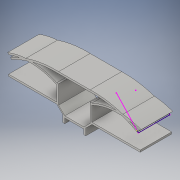
# Autodesk Inventor part: Test
Saved by Autodesk Inventor 2016 (Build 200138000, 138)
## iProperties
Created: 2015-09-24
Part Number: Test
Material: Generic
Document SubType Name: Modeling
Designer: fei
Density: 1 g/cm^3
Appearance: Default
Author: fei
Autodesk Inventor part; units mm, degrees
ref_plane "YZ Plane" through (0, 0, 0) normal (1, 0, 0) x (0, 1, 0)
ref_plane "XZ Plane" through (0, 0, 0) normal (0, 1, 0) x (-1, 0, 0)
ref_plane "XY Plane" through (0, 0, 0) normal (0, 0, 1) x (1, 0, 0)
sketch "Sketch1" plane through (0, 0, 0) normal (1, 0, 0) x (0, 1, 0)
  line L0 (38.1, 647.7) -> (-38.1, 647.7)
  line L1 (-38.1, 647.7) -> (-38.1, -647.7)
  line L2 (-38.1, -647.7) -> (38.1, -647.7)
  line L3 (38.1, -647.7) -> (38.1, 647.7)
  line L4 (0, 0) -> (420.0175, 0) construction
  point P0 (0, 647.7)
  dimension "d0" = 76.2
  dimension "d1" = 1295.4
  dimension "d2" = 647.7
  constraints: 10 end point, 2 horizontal, 2 parallel, 1 midpoint, 1 perpendicular, 1 vertical alignment
  measures "d0" distance of L1.end L2.end
  measures "d1" distance of L2.end L0.start
  measures "d2" distance between parallel lines of L0 L4
extrude "Extrusion1" add sketch "Sketch1" along normal blind 469.9
sketch "Sketch2" plane through (0, -38.1, -647.7) normal (0, -1, 0) x (1, 0, 0)
  line L0 (0, 0) -> (469.9, 0) projected
  line L1 (469.9, 1295.4) -> (393.7, 1295.4)
  line L2 (393.7, 1295.4) -> (393.7, 0)
  line L3 (393.7, 0) -> (469.9, 0)
  line L4 (469.9, 0) -> (469.9, 1295.4)
  point P0 (0, 647.7)
  dimension "d5" = 76.2
  constraints: 8 end point, 2 parallel, 1 horizontal, 1 perpendicular, 1 point on line
  measures "d5" distance of L2.end L0.end
extrude "Extrusion2" add sketch "Sketch2" along normal blind 203.2
sketch "Sketch3" plane through (0, 38.1, 647.7) normal (0, 1, 0) x (1, 0, 0)
  line L0 (469.9, 1295.4) -> (469.9, 0) projected
  line L1 (393.7, 0) -> (393.7, 1295.4) projected
  line L2 (469.9, 1295.4) -> (393.7, 1295.4)
  line L3 (393.7, 1295.4) -> (393.7, 0)
  line L4 (393.7, 0) -> (469.9, 0)
  line L5 (469.9, 0) -> (469.9, 1295.4)
  point P0 (0, 647.7)
  constraints: 8 end point, 2 parallel, 1 horizontal, 1 perpendicular
sketch "Sketch4" plane through (0, 0, 0) normal (0, 0, 1) x (1, 0, 0)
  line L0 (0, 38.1) -> (469.9, 38.1) projected
  line L1 (431.8, 38.1) -> (685.8, 292.1)
  point P0 (0, 0)
  dimension "d10" = 135
  dimension "d11" = 38.1
  dimension "d12" = 254
  constraints: 2 end point, 1 point on line
  measures "d10" angle of L0 L1
  measures "d11" distance of L0.end L1.start
  measures "d12" horizontal distance of L1.start L1.end
sweep "Sweep1" add profiles "Sketch3" path "Sketch4" path curves L1
sketch "Sketch5" plane through (647.7, 292.1, -647.7) normal (0, 1, 0) x (1, 0, 0)
  line L0 (76.2, -1295.4) -> (76.2, 0) projected
  line L1 (-254, -1295.4) -> (0, -1295.4) projected
  line L2 (76.2, 0) -> (0, 0)
  line L3 (0, 0) -> (0, -1295.4)
  line L4 (0, -1295.4) -> (76.2, -1295.4)
  line L5 (76.2, -1295.4) -> (76.2, 0)
  point P0 (-647.7, -647.7)
  constraints: 8 end point, 2 parallel, 1 horizontal, 1 perpendicular
extrude "Extrusion3" add sketch "Sketch5" along normal blind 76.2
sketch "Sketch6" plane through (723.9, 292.1, -647.7) normal (1, 0, 0) x (0, 0, -1)
  line L0 (-1295.4, 0) -> (-1295.4, 76.2) projected
  line L1 (0, -254) -> (0, 0) projected
  line L2 (-1295.4, 76.2) -> (0, 76.2)
  line L3 (0, 76.2) -> (0, 0)
  line L4 (0, 0) -> (-1295.4, 0)
  line L5 (-1295.4, 0) -> (-1295.4, 76.2)
  point P0 (-647.7, -292.1)
  constraints: 8 end point, 2 parallel, 1 horizontal, 1 perpendicular
extrude "Extrusion4" add sketch "Sketch6" along normal blind 1981.2
sketch "Sketch7" plane through (647.7, 368.3, -647.7) normal (0, 1, 0) x (1, 0, 0)
  line L0 (0, 0) -> (0, -1295.4) projected
  line L1 (0, 0) -> (76.2, 0)
  line L2 (76.2, 0) -> (76.2, -1295.4)
  line L3 (76.2, -1295.4) -> (0, -1295.4)
  line L4 (0, -1295.4) -> (0, 0)
  point P0 (-647.7, -647.7)
  dimension "d19" = 76.2
  constraints: 8 end point, 2 parallel, 1 horizontal, 1 perpendicular
  measures "d19" distance of L0.start L1.end
extrude "Extrusion5" add sketch "Sketch7" along normal blind 609.6
sketch "Sketch8" plane through (0, 0, 0) normal (0, 0, 1) x (1, 0, 0)
  line L0 (647.7, 977.9) -> (723.9, 977.9) projected
  arc A0 (2705.1, 1079.5) -> (685.8, 977.9) centre (1812.5424, -1298.512) ccw
  line L1 (723.9, 977.9) -> (2746.3916, 977.9) construction
  line L2 (723.9, 368.3) -> (2705.1, 368.3) construction
  line L3 (2705.1, 368.3) -> (2705.1, 1575.1367) construction
  point P0 (0, 0)
  dimension "d22" = 2540
  dimension "d23" = 101.6
  constraints: 4 end point, 2 point on circle, 1 centre point, 1 horizontal, 1 midpoint, 1 point on line, 1 vertical
  measures "d22" radius of A0
  measures "d23" distance from line of L1 A0.start
sketch "Sketch9" plane through (647.7, 977.9, -647.7) normal (0, 1, 0) x (1, 0, 0)
  line L0 (0, 0) -> (0, -1295.4) projected
  line L1 (-177.8, -1295.4) -> (76.2, -1295.4) projected
  line L2 (0, 0) -> (76.2, 0)
  line L3 (76.2, 0) -> (76.2, -1295.4)
  line L4 (76.2, -1295.4) -> (0, -1295.4)
  line L5 (0, -1295.4) -> (0, 0)
  point P0 (-647.7, -647.7)
  constraints: 8 end point, 2 parallel, 1 horizontal, 1 perpendicular
sketch "Sketch12" plane through (0, 0, 0) normal (1, 0, 0) x (0, 1, 0)
  line L0 (1487.2171, -647.7) -> (1411.0171, -647.7)
  line L1 (1411.0171, -647.7) -> (1411.0171, 647.7)
  line L2 (1411.0171, 647.7) -> (1487.2171, 647.7)
  line L3 (1487.2171, 647.7) -> (1487.2171, -647.7)
  line L4 (876.3, -647.7) -> (1157.0171, -647.7) construction
  line L5 (876.3, 647.7) -> (1157.0171, 647.7) construction
  line L6 (1157.0171, -647.7) -> (1157.0171, 647.7) construction
  point P0 (0, 0)
  point P1 (1005.7223, -647.7)
  point P2 (1005.7223, 647.7)
  dimension "d26" = 1295.4
  dimension "d27" = 76.2
  dimension "d28" = 254
  dimension "d29" = 647.7
  constraints: 10 end point, 2 parallel, 1 horizontal, 1 perpendicular, 1 vertical
  measures "d26" distance of L2.end L0.start
  measures "d27" distance of L0.start L0.end
  measures "d28" distance between parallel lines of L6 L1
  measures "d29" distance from line of point (0, 0) L0
extrude "Extrusion6" add sketch "Sketch12" along normal blind 647.7
sketch "Sketch13" plane through (0, 0, 0) normal (0, 0, 1) x (1, 0, 0)
  line L0 (2577.4706, 1005.7223) -> (2629.5294, 950.0777) projected
  line L1 (647.7, 1411.0171) -> (647.7, 1487.2171) projected
  arc A0 (2603.5, 977.9) -> (647.7, 1449.1171) centre (764.8444, -2359.0815) ccw
  point P0 (0, 0)
  dimension "d32" = 3810
  constraints: 2 midpoint, 2 point on circle, 1 centre point
  measures "d32" radius of A0
ref_plane "Work Plane2" through (2577.4706, 1005.7223, 647.7) normal (0.7302, 0.6832, 0) x (0, 0, -1)
sketch "Sketch14" plane through (2577.4706, 1005.7223, 647.7) normal (0.7302, 0.6832, 0) x (0, 0, -1)
  line L0 (0, -76.2) -> (0, 1241.2384) projected
  line L1 (0, -76.2) -> (1295.4, -76.2) projected
  line L2 (0, -0.6753) -> (1295.4, -0.6753)
  line L3 (1295.4, -0.6753) -> (1295.4, -76.2)
  line L4 (1295.4, -76.2) -> (0, -76.2)
  line L5 (0, -76.2) -> (0, -0.6753)
  point P0 (647.7, 1026.474)
  constraints: 8 end point, 2 parallel, 1 horizontal, 1 perpendicular, 1 point on line
sketch "Sketch15" plane through (647.7, 0, 0) normal (1, 0, 0) x (0, 0, -1)
  line L0 (647.7, 1487.2171) -> (-647.7, 1487.2171) projected
  line L1 (647.7, 1411.0171) -> (647.7, 1487.2171) projected
  line L2 (-647.7, 1487.2171) -> (647.7, 1487.2171)
  line L3 (647.7, 1487.2171) -> (647.7, 1411.0171)
  line L4 (647.7, 1411.0171) -> (-647.7, 1411.0171)
  line L5 (-647.7, 1411.0171) -> (-647.7, 1487.2171)
  point P0 (0, 0)
  constraints: 8 end point, 2 parallel, 1 horizontal, 1 perpendicular
sweep "Sweep3" add profiles "Sketch15" path "Sketch13" path curves A0
extrude "Extrusion7" add sketch "Sketch9" along normal blind 76.2
sketch "Sketch16" plane through (723.9, 368.3, 647.7) normal (1, 0, 0) x (0, 0, -1)
  line L0 (0, 0) -> (0, 685.8) projected
  line L1 (1295.4, 0) -> (1295.4, 685.8) projected
  line L2 (0, 685.8) -> (1295.4, 685.8)
  line L3 (1295.4, 685.8) -> (1295.4, 609.6)
  line L4 (1295.4, 609.6) -> (0, 609.6)
  line L5 (0, 609.6) -> (0, 685.8)
  point P0 (647.7, -368.3)
  dimension "d37" = 76.2
  constraints: 8 end point, 2 parallel, 1 horizontal, 1 perpendicular, 1 point on line
  measures "d37" distance of L3.end L1.end
sweep "Sweep4" add profiles "Sketch16" path "Sketch8" path curves A0
mirror "Mirror1" about plane through (0, 0, 0) normal (1, 0, 0) of "Extrusion1", "Extrusion2", "Sweep1", "Extrusion3", "Extrusion4", "Extrusion5", "Extrusion6", "Sweep3", "Extrusion7", "Sweep4"
body "Solid1"
